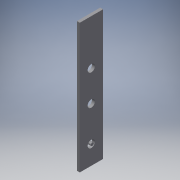
# Autodesk Inventor part: Gear-wall-motor-side
Saved by Autodesk Inventor 2017 (Build 210142000, 142)
## iProperties
Created: 2017-11-22
Part Number: Gear-wall-motor-side
Material: Generic
Document SubType Name: Modeling
Designer: julie
Density: 1 g/cm^3
Appearance: Default
Author: julie
Autodesk Inventor part; units mm, degrees
ref_plane "YZ Plane" through (0, 0, 0) normal (1, 0, 0) x (0, 1, 0)
ref_plane "XZ Plane" through (0, 0, 0) normal (0, 1, 0) x (-1, 0, 0)
ref_plane "XY Plane" through (0, 0, 0) normal (0, 0, 1) x (1, 0, 0)
sketch "Sketch1" plane through (0, 0, 0) normal (1, 0, 0) x (0, 1, 0)
  line L0 (0, 0) -> (16, 0)
  line L1 (16, 0) -> (16, -89)
  line L2 (16, -89) -> (0, -89)
  line L3 (0, -89) -> (0, 0)
  dimension "d0" = 16
  dimension "d1" = 89
  constraints: 8 end point, 2 parallel, 1 horizontal, 1 perpendicular
  measures "d0" distance of L1.end L2.end
  measures "d1" distance of L0.end L1.end
extrude "Extrusion1" add sketch "Sketch1" along normal blind 2
sketch "Sketch2" plane through (2, 0, 0) normal (1, 0, 0) x (0, 0, -1)
  circle A0 centre (76.5, 8.5) radius 1 projected
  circle A1 centre (52, 7.8652) radius 2.5 projected
  circle A2 centre (31, 7.8652) radius 2.5 projected
  circle A3 centre (31, 7.8652) radius 2.5
  circle A4 centre (52, 7.8652) radius 2.5
  circle A5 centre (76.1279, 7.6338) radius 2.5 projected
  line L0 (31, 7.8652) -> (88.1089, 7.8652) construction
  circle A6 centre (76, 7.8652) radius 2.5
  point P0 (0, 0)
  dimension "d4" = 5
  dimension "d5" = 5
  dimension "d6" = 5
  dimension "d9" = 21
  dimension "d10" = 24
  constraints: 3 centre point, 2 coincident, 2 end point, 1 horizontal, 1 point on line
  measures "d4" diameter of A3
  measures "d5" diameter of A4
  measures "d6" diameter of A6
  measures "d9" distance of A1.centre A2.centre
  measures "d10" distance of A6.centre A1.centre
extrude "Extrusion2" cut sketch "Sketch2" against normal blind 2 contours A1 | A2 | A6 A5 | A5 A6 picked at (74.9617, 6.4955) picked at (74.7573, 9.9128)
body "Solid1"
